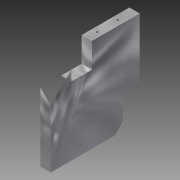
# Autodesk Inventor part: CavitySplitter
Saved by Autodesk Inventor 2014 (Build 180170000, 170)
## iProperties
Created: 2015-04-19
Part Number: CavitySplitter
Material: Generic
Document SubType Name: Modeling
Designer: Owner
Density: 1 g/cm^3
Appearance: Aluminum - Polished
Author: Owner
Autodesk Inventor part; units mm, degrees
ref_plane "YZ Plane" through (0, 0, 0) normal (1, 0, 0) x (0, 1, 0)
ref_plane "XZ Plane" through (0, 0, 0) normal (0, 1, 0) x (-1, 0, 0)
ref_plane "XY Plane" through (0, 0, 0) normal (0, 0, 1) x (1, 0, 0)
sketch "Sketch1" plane through (0, 0, 0) normal (1, 0, 0) x (0, 1, 0)
  line L0 (-65.0537, 22.225) -> (-7.9037, 22.225)
  line L1 (-7.9037, 22.225) -> (-7.9037, -22.225)
  line L2 (-7.9037, -22.225) -> (-65.0537, -22.225)
  line L3 (-65.0537, -22.225) -> (-65.0537, 22.225)
  line L4 (-7.9037, -3.175) -> (-23.1437, -3.175)
  line L5 (-23.1437, -3.175) -> (-23.1437, 9.525)
  line L6 (-23.1437, 9.525) -> (-7.9037, 9.525)
  line L7 (-7.9037, 9.525) -> (-7.9037, -3.175)
  line L8 (-7.9037, -22.225) -> (-46.0037, -22.225)
  line L9 (-46.0037, -22.225) -> (-46.0037, -32.385)
  line L10 (-46.0037, -32.385) -> (-7.9037, -32.385)
  line L11 (-7.9037, -32.385) -> (-7.9037, -22.225)
  point P0 (0, 0)
  dimension "d2" = 57.15
  dimension "d3" = 44.45
  dimension "d4" = 15.24
  dimension "d5" = 12.7
  dimension "d7" = 10.16
  dimension "d8" = 38.1
  dimension "d10" = 19.05
  constraints: 24 end point, 6 parallel, 3 horizontal, 3 perpendicular, 1 point on line
  measures "d2" distance of L0.start L0.end
  measures "d3" distance of L0.end L1.end
  measures "d4" distance of L5.end L6.end
  measures "d5" distance of L4.end L5.end
  measures "d7" distance of L10.end L1.end
  measures "d8" distance of L9.end L10.end
  measures "d10" distance between parallel lines of L2 L4
extrude "Extrusion1" add sketch "Sketch1" along normal blind 6.35 contours L0 L1 L6 L5 L4 L2 L3 | L2 L11 L10 L9
sketch "Sketch2" plane through (0, -65.0537, -22.225) normal (0, -1, 0) x (1, 0, 0)
  point P0 (3.175, 6.35)
hole "Hole1" at (3.175, -65.0537, -15.875) direction (0, 1, 0) diameter 1.1811 depth 4.699 tip angle 120 thread size "0-80 UNF" class "2B" standard "ANSI Unified Screw Threads"
pattern_linear "Rectangular Pattern1" count 3 spacing 12.7 along (0, 0, 1) of "Hole1"
sketch "Sketch3" plane through (0, -7.9037, -3.175) normal (0, 1, 0) x (1, 0, 0)
  point P0 (3.175, 6.35)
hole "Hole3" at (3.175, -7.9037, -9.525) direction (0, -1, 0) diameter 1.1811 depth 4.699 tip angle 120 thread size "0-80 UNF" class "2B" standard "ANSI Unified Screw Threads"
pattern_linear "Rectangular Pattern2" count 2 spacing 25.4 along (0, 0, 1) of "Hole3"
pattern_linear "Rectangular Pattern3" count 2 spacing 12.7 along (0, 0, -1) of "Hole3"
sketch "Sketch4" plane through (0, 0, 0) normal (-1, 0, 0) x (0, 0, 1)
  point P0 (-10.16, -49.1837)
hole "Hole5" at (0, -49.1837, -10.16) direction (1, 0, 0) diameter 3.4544 depth 6.35
sketch "Sketch5" plane through (0, 0, 0) normal (-1, 0, 0) x (0, 0, 1)
  point P0 (-16.51, -26.9587)
hole "Hole7" at (0, -26.9587, -16.51) direction (1, 0, 0) diameter 3.4544 depth 6.35
body "Solid1"
